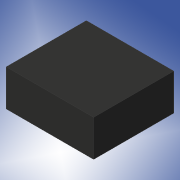
# Autodesk Inventor part: ExpertPower EXP12180 Battery
Saved by Autodesk Inventor 2017 SP1 (Build 210196100, 196)
## iProperties
Created: 2017-08-08
Part Number: ExpertPower EXP12180 Battery
Material: PC/ABS Plastic
Document SubType Name: Modeling
Designer: Zach
Density: 0.357273 g/cm^3
Appearance: Rubber - Black
Catalog Web Link: https://www.amazon.com/gp/product/B00A82A3RK/ref=oh_aui_detailpage_o05_s02?ie=UTF8&th=1
Author: Zach
Autodesk Inventor part; units mm, degrees
ref_plane "YZ Plane" through (0, 0, 0) normal (1, 0, 0) x (0, 1, 0)
ref_plane "XZ Plane" through (0, 0, 0) normal (0, 1, 0) x (-1, 0, 0)
ref_plane "XY Plane" through (0, 0, 0) normal (0, 0, 1) x (1, 0, 0)
sketch "Sketch1" plane through (0, 0, 0) normal (0, 0, 1) x (1, 0, 0)
  line L0 (0, 0) -> (180, 0)
  line L1 (180, 0) -> (180, 75)
  line L2 (180, 75) -> (0, 75)
  line L3 (0, 75) -> (0, 0)
  dimension "d0" = 180
  dimension "d1" = 75
  constraints: 8 end point, 2 parallel, 1 horizontal, 1 perpendicular
  measures "d0" distance of L2.end L1.end
  measures "d1" distance of L1.end L0.end
extrude "Extrusion1" add sketch "Sketch1" along normal blind 165
body "Solid1"
